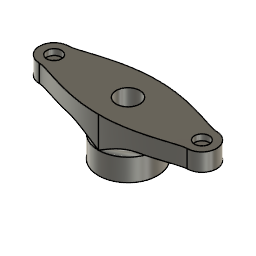
HighRocker_v5 (Autodesk Fusion 360 design; units mm, degrees)
Autodesk Fusion 360 part; units mm, degrees
sketch "Sketch1" plane through (0, 0, 0) normal (0, 0, 1) x (1, 0, 0)
  line L0 (-1.2354, -2.9557) -> (-0.9535, -3.0583)
  line L1 (2.8181, 1.7189) -> (3.2903, 2.2747)
  line L2 (-2.8463, -1.4701) -> (-2.6963, -1.7299)
  line L3 (3.2361, -0.6514) -> (3.2637, -0.4947)
  line L4 (-3.6151, -1.7121) -> (-2.8976, -1.5811)
  line L5 (-2.0603, 2.5791) -> (-2.1821, 2.4768)
  line L6 (-2.0603, -2.5791) -> (-2.3138, -3.2628)
  line L7 (2.6963, 1.7299) -> (3.1639, 2.2804)
  line L8 (-2.8976, -1.5811) -> (-2.8181, -1.7189)
  line L9 (3.1253, -0.7034) -> (3.1774, -0.408)
  line L10 (3.1774, -0.408) -> (3.8894, -0.2868)
  line L11 (-2.1718, -2.3549) -> (-1.942, -2.5478)
  arc A0 (1.6963, -3.5118) -> (2.1931, -3.2249) centre (0, 0) ccw
  line L12 (1.0539, -3.1282) -> (1.2034, -3.0738)
  line L13 (-3.5568, -1.5998) -> (-2.8463, -1.4701)
  arc A1 (-3.9826, 0.3724) -> (-3.9826, -0.3724) centre (0, 0) ccw
  arc A2 (3.9826, -0.3724) -> (3.9826, 0.3724) centre (0, 0) ccw
  arc A3 (0.3929, -3.8802) -> (0.9579, -3.7805) centre (0, 0) ccw
  line L14 (1.942, 2.5478) -> (2.1931, 3.2249)
  line L15 (3.2361, 0.6514) -> (3.8698, 1.0122)
  arc A4 (-2.3138, -3.2628) -> (-1.6688, -3.6353) centre (0, 0) ccw
  line L16 (3.6151, 1.7121) -> (2.8976, 1.5811)
  line L17 (-3.8894, -0.2868) -> (-3.1774, -0.408)
  arc A5 (1.6688, -3.6353) -> (2.3138, -3.2628) centre (0, 0) ccw
  line L18 (1.2034, -3.0738) -> (1.6688, -3.6353)
  line L19 (-2.8115, -2.8453) -> (-2.1821, -2.4768)
  line L20 (-2.1821, -2.4768) -> (-2.0603, -2.5791)
  line L21 (2.1821, 2.4768) -> (2.0603, 2.5791)
  line L22 (-1.942, -2.5478) -> (-2.1931, -3.2249)
  line L23 (1.2354, -2.9557) -> (1.6963, -3.5118)
  line L24 (3.1639, -2.2804) -> (2.6963, -1.7299)
  line L25 (3.1774, 0.408) -> (3.1253, 0.7034)
  line L26 (-3.2361, -0.6514) -> (-3.8698, -1.0122)
  line L27 (-1.2354, 2.9557) -> (-1.6963, 3.5118)
  line L28 (-0.15, 3.2) -> (-0.3929, 3.8802)
  line L29 (-0.0795, 3.3) -> (-0.3248, 3.9868)
  line L30 (2.8463, -1.4701) -> (3.5568, -1.5998)
  arc A6 (-3.5568, 1.5998) -> (-3.753, 1.0607) centre (0, 0) ccw
  line L31 (2.1718, -2.3549) -> (2.7951, -2.7198)
  line L32 (-0.3929, -3.8802) -> (-0.15, -3.2)
  line L33 (-1.6963, -3.5118) -> (-1.2354, -2.9557)
  line L34 (3.8894, 0.2868) -> (3.1774, 0.408)
  line L35 (2.8976, 1.5811) -> (2.8181, 1.7189)
  line L36 (1.0539, 3.1282) -> (1.0583, 3.8574)
  arc A7 (3.753, 1.0607) -> (3.5568, 1.5998) centre (0, 0) ccw
  line L37 (-0.15, -3.2) -> (0.15, -3.2)
  line L38 (3.9826, 0.3724) -> (3.2637, 0.4947)
  arc A8 (2.8115, -2.8453) -> (3.2903, -2.2747) centre (0, 0) ccw
  line L39 (-1.0539, -3.1282) -> (-1.0583, -3.8574)
  line L40 (-2.8976, 1.5811) -> (-3.6151, 1.7121)
  arc A9 (2.7951, -2.7198) -> (3.1639, -2.2804) centre (0, 0) ccw
  line L41 (-2.6963, -1.7299) -> (-3.1639, -2.2804)
  line L42 (0.9579, -3.7805) -> (0.9535, -3.0583)
  line L43 (-1.6688, -3.6353) -> (-1.2034, -3.0738)
  arc A10 (-3.753, -1.0607) -> (-3.5568, -1.5998) centre (0, 0) ccw
  line L44 (2.0603, -2.5791) -> (2.1821, -2.4768)
  line L45 (-0.0795, -3.3) -> (0.0795, -3.3)
  line L46 (-3.2637, -0.4947) -> (-3.2361, -0.6514)
  arc A11 (2.3138, 3.2628) -> (1.6688, 3.6353) centre (0, 0) ccw
  line L47 (-3.1253, -0.7034) -> (-3.753, -1.0607)
  arc A12 (-3.8698, -1.0122) -> (-3.6151, -1.7121) centre (0, 0) ccw
  line L48 (3.1253, 0.7034) -> (3.753, 1.0607)
  line L49 (-1.2034, -3.0738) -> (-1.0539, -3.1282)
  line L50 (2.8976, -1.5811) -> (3.6151, -1.7121)
  line L51 (-2.8181, -1.7189) -> (-3.2903, -2.2747)
  arc A13 (-3.2903, -2.2747) -> (-2.8115, -2.8453) centre (0, 0) ccw
  line L52 (-3.1774, 0.408) -> (-3.8894, 0.2868)
  line L53 (0.0795, -3.3) -> (0.3248, -3.9868)
  line L54 (0.9535, -3.0583) -> (1.2354, -2.9557)
  line L55 (2.1821, -2.4768) -> (2.8115, -2.8453)
  line L56 (3.5568, 1.5998) -> (2.8463, 1.4701)
  arc A14 (3.8698, 1.0122) -> (3.6151, 1.7121) centre (0, 0) ccw
  line L57 (3.2903, -2.2747) -> (2.8181, -1.7189)
  arc A15 (0.9579, 3.7805) -> (0.3929, 3.8802) centre (0, 0) ccw
  arc A16 (-3.1639, -2.2804) -> (-2.7951, -2.7198) centre (0, 0) ccw
  line L58 (-3.9826, -0.3724) -> (-3.2637, -0.4947)
  arc A17 (-2.1931, -3.2249) -> (-1.6963, -3.5118) centre (0, 0) ccw
  line L59 (2.8463, 1.4701) -> (2.6963, 1.7299)
  line L60 (1.942, -2.5478) -> (2.1718, -2.3549)
  line L61 (-2.1931, 3.2249) -> (-1.942, 2.5478)
  line L62 (-0.9535, -3.0583) -> (-0.9579, -3.7805)
  arc A18 (-2.7951, 2.7198) -> (-3.1639, 2.2804) centre (0, 0) ccw
  line L63 (-3.1774, -0.408) -> (-3.1253, -0.7034)
  line L64 (3.8698, -1.0122) -> (3.2361, -0.6514)
  line L65 (2.3138, -3.2628) -> (2.0603, -2.5791)
  line L66 (0.15, -3.2) -> (0.3929, -3.8802)
  arc A19 (3.5568, -1.5998) -> (3.753, -1.0607) centre (0, 0) ccw
  line L67 (3.2637, 0.4947) -> (3.2361, 0.6514)
  line L68 (0.9535, 3.0583) -> (0.9579, 3.7805)
  line L69 (-2.1718, 2.3549) -> (-2.7951, 2.7198)
  line L70 (-0.3248, -3.9868) -> (-0.0795, -3.3)
  arc A20 (-0.3929, 3.8802) -> (-0.9579, 3.7805) centre (0, 0) ccw
  line L71 (3.2637, -0.4947) -> (3.9826, -0.3724)
  arc A21 (-0.3248, 3.9868) -> (-1.0583, 3.8574) centre (0, 0) ccw
  arc A22 (3.6151, -1.7121) -> (3.8698, -1.0122) centre (0, 0) ccw
  arc A23 (-0.9579, -3.7805) -> (-0.3929, -3.8802) centre (0, 0) ccw
  line L72 (2.6963, -1.7299) -> (2.8463, -1.4701)
  line L73 (-3.8698, 1.0122) -> (-3.2361, 0.6514)
  line L74 (2.0603, 2.5791) -> (2.3138, 3.2628)
  line L75 (-3.2903, 2.2747) -> (-2.8181, 1.7189)
  arc A24 (-1.6688, 3.6353) -> (-2.3138, 3.2628) centre (0, 0) ccw
  line L76 (-3.1253, 0.7034) -> (-3.1774, 0.408)
  line L77 (-3.2361, 0.6514) -> (-3.2637, 0.4947)
  arc A25 (-3.6151, 1.7121) -> (-3.8698, 1.0122) centre (0, 0) ccw
  arc A26 (-2.8115, 2.8453) -> (-3.2903, 2.2747) centre (0, 0) ccw
  line L78 (2.1718, 2.3549) -> (1.942, 2.5478)
  line L79 (-2.6963, 1.7299) -> (-2.8463, 1.4701)
  arc A27 (1.0583, 3.8574) -> (0.3248, 3.9868) centre (0, 0) ccw
  line L80 (0.3929, 3.8802) -> (0.15, 3.2)
  line L81 (-3.1639, 2.2804) -> (-2.6963, 1.7299)
  line L82 (2.7951, 2.7198) -> (2.1718, 2.3549)
  line L83 (2.8115, 2.8453) -> (2.1821, 2.4768)
  line L84 (-1.0539, 3.1282) -> (-1.2034, 3.0738)
  line L85 (1.2354, 2.9557) -> (0.9535, 3.0583)
  line L86 (0.15, 3.2) -> (-0.15, 3.2)
  line L87 (-1.0583, 3.8574) -> (-1.0539, 3.1282)
  line L88 (0.3248, 3.9868) -> (0.0795, 3.3)
  arc A28 (2.1931, 3.2249) -> (1.6963, 3.5118) centre (0, 0) ccw
  arc A29 (3.1639, 2.2804) -> (2.7951, 2.7198) centre (0, 0) ccw
  line L89 (-2.8463, 1.4701) -> (-3.5568, 1.5998)
  line L90 (1.6963, 3.5118) -> (1.2354, 2.9557)
  arc A30 (3.2903, 2.2747) -> (2.8115, 2.8453) centre (0, 0) ccw
  line L91 (-0.9579, 3.7805) -> (-0.9535, 3.0583)
  line L92 (1.6688, 3.6353) -> (1.2034, 3.0738)
  line L93 (-3.2637, 0.4947) -> (-3.9826, 0.3724)
  line L94 (-3.753, 1.0607) -> (-3.1253, 0.7034)
  line L95 (-1.942, 2.5478) -> (-2.1718, 2.3549)
  line L96 (1.2034, 3.0738) -> (1.0539, 3.1282)
  arc A31 (-1.6963, 3.5118) -> (-2.1931, 3.2249) centre (0, 0) ccw
  line L97 (0.0795, 3.3) -> (-0.0795, 3.3)
  line L98 (-2.8181, 1.7189) -> (-2.8976, 1.5811)
  line L99 (-2.1821, 2.4768) -> (-2.8115, 2.8453)
  line L100 (-1.2034, 3.0738) -> (-1.6688, 3.6353)
  line L101 (-0.9535, 3.0583) -> (-1.2354, 2.9557)
  line L102 (-2.3138, 3.2628) -> (-2.0603, 2.5791)
  line L103 (-2.7951, -2.7198) -> (-2.1718, -2.3549)
  line L104 (2.8181, -1.7189) -> (2.8976, -1.5811)
  circle A32 centre (0, 0) radius 1.5
  arc A33 (3.8894, -0.2868) -> (3.8894, 0.2868) centre (0, 0) ccw
  arc A34 (-1.0583, -3.8574) -> (-0.3248, -3.9868) centre (0, 0) ccw
  arc A35 (-3.8894, 0.2868) -> (-3.8894, -0.2868) centre (0, 0) ccw
  line L105 (2.1931, -3.2249) -> (1.942, -2.5478)
  arc A36 (0.3248, -3.9868) -> (1.0583, -3.8574) centre (0, 0) ccw
  line L106 (3.753, -1.0607) -> (3.1253, -0.7034)
  line L107 (1.0583, -3.8574) -> (1.0539, -3.1282)
  circle A37 centre (0, 0) radius 10
  line L108 (30, -5) -> (-30, -5)
  line L109 (-30, -5) -> (-30, 5)
  line L110 (-30, 5) -> (30, 5)
  line L111 (30, 5) -> (30, -5)
  line L112 (30, -5) -> (-30, 5) construction
  line L113 (-30, -5) -> (30, 5) construction
  line L114 (25, 0) -> (-25, 0) construction
  circle A38 centre (-25, 0) radius 0.5
  circle A39 centre (25, 0) radius 0.5
  circle A40 centre (-25, 0) radius 5
  circle A41 centre (25, 0) radius 5
  spline S0 degree 5 poles (-25, 5) (-24.6986, 5) (-23.9176, 5.1002) (-22.2111, 5.5513) (-18.9203, 6.6553) (-13.4244, 8.3447) (-6.9604, 9.7247) (0, 10.2671) (6.9604, 9.7247) (13.4244, 8.3447) (18.9203, 6.6553) (22.2111, 5.5513) (23.9176, 5.1002) (24.6986, 5) (25, 5) knots 0 0 0 0 0 0 0.1 0.2 0.3 0.4 0.5 0.6 0.7 0.8 0.9 1 1 1 1 1 1
  spline S1 degree 5 poles (-25, -5) (-24.6986, -5) (-23.9176, -5.1002) (-22.2111, -5.5513) (-18.9203, -6.6553) (-13.4244, -8.3447) (-6.9604, -9.7247) (0, -10.2671) (6.9604, -9.7247) (13.4244, -8.3447) (18.9203, -6.6553) (22.2111, -5.5513) (23.9176, -5.1002) (24.6986, -5) (25, -5) knots 0 0 0 0 0 0 0.1 0.2 0.3 0.4 0.5 0.6 0.7 0.8 0.9 1 1 1 1 1 1
  line L115 (-26.5, 5) -> (-23.5, 5)
  line L116 (23.5, 5) -> (26.5, 5)
  line L117 (-26.5, -5) -> (-23.5, -5)
  line L118 (23.5, -5) -> (26.5, -5)
  circle A42 centre (-25, 0) radius 2.5
  circle A43 centre (25, 0) radius 2.5
  point P0 (0, 10)
  point P1 (0, -10)
  dimension "d1" = 0.1
  dimension "d2" = 3
  dimension "d3" = 20
  dimension "d4" = 60
  dimension "d5" = 10
  dimension "d6" = 50
  dimension "d7" = 1
  dimension "d8" = 1
  dimension "d15" = 5
  dimension "d16" = 5
  constraint concentric A0 A37
  constraint horizontal L108
  constraint perpendicular L108 L109
  constraint parallel L108 L110
  constraint parallel L109 L111
  constraint coincident L112 A0.centre
  constraint coincident L113 A0.centre
  constraint coincident A0.centre A1.centre
  constraint midpoint L114 A0.centre
  constraint horizontal L114
  constraint coincident L114.end A38.centre
  constraint coincident L114.start A39.centre
  constraint concentric A38 A40
  constraint tangent L109 A40
  constraint concentric A39 A41
  constraint tangent L111 A41
  constraint coincident L110 S0.start
  constraint coincident A37 P0
  constraint coincident A41 S0.end
  constraint coincident L110 S0.end
  constraint midpoint S0.start L115
  constraint midpoint S0.end L116
  constraint symmetric L114 S0.start S1.start
  constraint symmetric L114 P0 P1
  constraint symmetric L114 S0.end S1.end
  constraint symmetric L114 L115.start L117.start
  constraint symmetric L114 L115.end L117.end
  constraint symmetric L114 L116.start L118.start
  constraint symmetric L114 L116.end L118.end
  constraint coincident L110 L116.end
  constraint coincident L110 L115.end
  constraint concentric A40 A42
  constraint concentric A39 A43
  measures "d2" diameter of A32
  measures "d3" diameter of A37
  measures "d4" distance of L109.end L110.end
  measures "d5" distance of L108.end L109.end
  measures "d6" distance of L114.start L114.end
  measures "d7" diameter of A38
  measures "d8" diameter of A39
  measures "d15" diameter of A42
  measures "d16" diameter of A43
extrude "Extrude1" add sketch "Sketch1" along normal blind 6 contours A37 L108 L110 | A37 L108 L110 A41 L116 L118 | A37 L110 | A37 L110 S0 L116 | A37 L108 S1 L118 | A37 L108 | A37 L110 S0 L115 | A37 L108 L110 A40 L115 L117 | A37 L108 S1 L117 | A40 | A41 | A42 | A43
extrude "Extrude2" add sketch "Sketch1" against normal blind 12 contours A37 L108 L110 | A37 L110 | A37 L108
fillet "Fillet1" radius 4.5 2 edges at (10, 0, 0) (-10, 0, 0)
extrude "Extrude3" cut sketch "Sketch1" along normal blind 2 from surface at 4 contours A42 | A43
extrude "Extrude4" add sketch "Sketch1" along normal blind 6 and the other way blind 6 contours L0 L2 L7 L9 L10 L11 A0 L13 A3 L14 L17 L22 L23 L24 L25 L27 L28 L30 A6 L31 L32 L33 L34 A7 L37 A9 L41 L42 A10 L47 L48 L52 L54 L56 A15 A16 A17 L59 L60 L61 L62 A18 L63 L66 A19 L68 L69 A20 A23 L72 L76 L78 L79 L80 L81 L82 L85 L86 A28 A29 L89 L90 L91 L94 L95 A31 L101 L103 A33 A35 L105 L106 | L1 L3 L4 L5 L6 L8 L12 A1 A2 L15 A4 L16 A5 L18 L19 L20 L21 L26 L29 L35 L36 L38 A8 L39 L40 L43 L44 L45 L46 A11 A12 L49 L50 L51 A13 L53 L55 A14 L57 L58 L64 L65 L67 L70 L71 A21 A22 L73 L74 L75 A24 L77 A25 A26 A27 L83 L84 L87 L88 A30 L92 L93 L96 L97 L98 L99 L100 L102 L104 A34 A36 L107
hole "Hole1" at (0, 0, 6) direction (0, 0, -1) diameter 8 depth 8 tip angle 180
equation "d22 = 12.00 mm - 6 mm"
